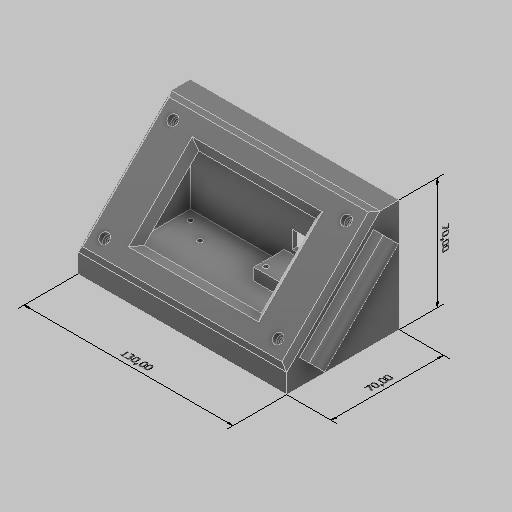
# Autodesk Inventor part: CASE - IHM
Saved by Autodesk Inventor 2025.2 (Build 292293000, 293)
## iProperties
Created: 2024-09-22
Part Number: CASE - IHM
Material: Genérico
Document SubType Name: Modeling
Designer: phmca
Density: 1 g/cm^3
Appearance: Suave - Preto
Author: phmca
Autodesk Inventor part; units mm, degrees
ref_plane "YZ Plane" through (0, 0, 0) normal (1, 0, 0) x (0, 1, 0)
ref_plane "XZ Plane" through (0, 0, 0) normal (0, 1, 0) x (-1, 0, 0)
sketch "Esboço1" plane through (0, 0, 0) normal (0, 1, 0) x (-1, 0, 0)
  line L0 (65, 35) -> (-65, 35)
  line L1 (-65, 35) -> (-65, -35)
  line L2 (-65, -35) -> (65, -35)
  line L3 (65, -35) -> (65, 35)
  point P0 (0, 0)
  dimension "d0" = 130
  dimension "d1" = 65
  dimension "d2" = 70
  dimension "d3" = 35
  constraints: 8 end point, 2 parallel, 1 horizontal, 1 perpendicular
  measures "d0" distance of L1.end L2.end
  measures "d1" distance from line of L3 point (0, 0)
  measures "d2" distance of L0.end L1.end
  measures "d3" distance from line of point (0, 0) L2
extrude "Extrusão1" add sketch "Esboço1" along normal blind 3
sketch "Esboço2" plane through (0, 3, 0) normal (0, 1, 0) x (1, 0, 0)
  line L0 (65, -35) -> (65, 35) projected
  line L1 (65, 35) -> (-65, 35) projected
  line L2 (-65, 35) -> (-65, -35) projected
  line L3 (-65, -35) -> (65, -35) projected
  line L4 (-62, 32) -> (62, 32)
  line L5 (62, 32) -> (62, -32)
  line L6 (62, -32) -> (-62, -32)
  line L7 (-62, -32) -> (-62, 32)
  point P0 (0, 0)
  dimension "d6" = 3
  dimension "d7" = 3
  dimension "d8" = 3
  dimension "d9" = 3
  constraints: 8 end point, 2 parallel, 1 horizontal, 1 perpendicular
  measures "d6" distance between parallel lines of L1 L4
  measures "d7" distance between parallel lines of L3 L6
  measures "d8" distance between parallel lines of L2 L7
  measures "d9" distance between parallel lines of L0 L5
extrude "Extrusão2" add sketch "Esboço2" along normal blind 67
sketch "Esboço3" plane through (-62, 3, 32) normal (1, 0, 0) x (0, 0, -1)
  line L0 (64, 0) -> (0, 0) projected
  line L1 (64, 0) -> (64, 67) projected
  line L2 (0, 67) -> (64, 67) projected
  line L3 (0, 0) -> (0, 67) projected
  line L4 (0, 64) -> (64, 64)
  point P0 (32, -3)
  dimension "d12" = 3
  constraints: 2 end point, 2 point on line, 1 perpendicular
  measures "d12" distance between parallel lines of L2 L4
extrude "Extrusão3" add sketch "Esboço3" along normal up to surface (124 mm away) contours L4 L3 L2 L1
sketch "Esboço4" plane through (65, 0, 35) normal (1, 0, 0) x (0, 0, -1)
  line L0 (0, 0) -> (0, 70) projected
  line L1 (0, 12) -> (58, 70)
  line L2 (70, 70) -> (0, 70) projected
  line L3 (0, 12) -> (0, 0) construction
  line L4 (58, 70) -> (70, 70) construction
  line L5 (67, 67) -> (3, 67) projected
  line L6 (70, 0) -> (70, 70) projected
  line L7 (58, 70) -> (70, 70)
  line L8 (0, 12) -> (0, 0)
  line L9 (0, 0) -> (70, 0) projected
  point P0 (35, 0)
  point P1 (55, 67)
  dimension "d15" = 45
  dimension "d20" = 3
  dimension "d21" = 4.2426
  dimension "d160" = 12
  dimension "d161" = 12
  constraints: 10 end point, 4 point on line, 3 collinear, 1 horizontal
  measures "d15" angle of L0 L1
  measures "d20" horizontal distance of L1.end point (55, 67)
  measures "d21" distance of L1.end point (55, 67)
  measures "d160" distance from line of L6 L1.end
  measures "d161" distance from line of L9 L1.start
extrude "Extrusão4" cut sketch "Esboço4" against normal up to surface (130 mm away) contours L0 L2 L1
sketch "Esboço6" plane through (-65, 12, 35) normal (0, 0.7071068, 0.7071068) x (1, 0, 0)
  line L0 (127, 77.7817) -> (3, 77.7817) projected
  line L1 (3, 77.7817) -> (3, 4.2426) projected
  line L2 (3, 4.2426) -> (127, 4.2426) projected
  line L3 (127, 4.2426) -> (127, 77.7817) projected
  line L4 (3, 77.7817) -> (11, 77.7817)
  line L5 (11, 77.7817) -> (11, 69.7817)
  line L6 (11, 69.7817) -> (3, 69.7817)
  line L7 (3, 69.7817) -> (3, 77.7817)
  line L8 (127, 77.7817) -> (119, 77.7817)
  line L9 (119, 77.7817) -> (119, 69.7817)
  line L10 (119, 69.7817) -> (127, 69.7817)
  line L11 (127, 69.7817) -> (127, 77.7817)
  line L12 (3, 4.2426) -> (11, 4.2426)
  line L13 (11, 4.2426) -> (11, 12.2426)
  line L14 (11, 12.2426) -> (3, 12.2426)
  line L15 (3, 12.2426) -> (3, 4.2426)
  line L16 (127, 4.2426) -> (119, 4.2426)
  line L17 (119, 4.2426) -> (119, 12.2426)
  line L18 (119, 12.2426) -> (127, 12.2426)
  line L19 (127, 12.2426) -> (127, 4.2426)
  point P0 (65, 16.2635)
  point P1 (119, 77.7817)
  point P2 (3, 12.2426)
  point P3 (11, 4.2426)
  point P4 (3, 69.7817)
  dimension "d31" = 8
  dimension "d32" = 8
  dimension "d33" = 8
  dimension "d34" = 8
  dimension "d35" = 8
  dimension "d36" = 8
  dimension "d37" = 8
  dimension "d38" = 8
  constraints: 32 end point, 8 parallel, 4 horizontal, 4 perpendicular
  measures "d31" distance of L5.end L6.end
  measures "d32" distance of L4.end L5.end
  measures "d33" distance of L10.end L9.end
  measures "d34" distance of L9.end L8.end
  measures "d35" distance of L14.end L13.end
  measures "d36" distance of L13.end L12.end
  measures "d37" distance of L17.end L18.end
  measures "d38" distance of L16.end L17.end
extrude "Extrusão6" [suppressed]
sketch "Esboço7" plane through (62, 3, -32) normal (-1, 0, 0) x (0, 0, 1)
  line L0 (64, 12) -> (12, 64) projected
  line L1 (12, 64) -> (0, 64) projected
  line L2 (0, 0) -> (0, 64) projected
  line L3 (64, 0) -> (0, 0) projected
  line L4 (64, 0) -> (64, 12) projected
  line L5 (12, 52.6863) -> (6.3431, 52.6863)
  line L6 (6.3431, 52.6863) -> (6.3431, 64)
  line L7 (58.3431, -13.6569) -> (65.4142, -13.6569)
  line L8 (58.3431, -13.6569) -> (52.6863, -13.6569)
  line L9 (52.6863, -13.6569) -> (52.6863, 2)
  point P0 (32, -3)
  point P1 (54, 6.3431)
  constraints: 10 end point, 3 horizontal, 2 perpendicular, 1 point on line
extrude "Extrusão7" [suppressed]
fillet "Arredondamento2" [suppressed]
sketch "Esboço8" plane through (62, 3, -32) normal (-1, 0, 0) x (0, 0, 1)
  line L0 (64, 12) -> (12, 64) projected
  line L1 (12, 64) -> (0, 64) projected
  line L2 (0, 0) -> (0, 64) projected
  line L3 (64, 0) -> (0, 0) projected
  line L4 (64, 0) -> (64, 12) projected
  line L5 (58.3431, 6.3431) -> (64, 6.3431)
  line L6 (6.3431, 58.3431) -> (6.3431, 64)
  point P0 (32, -3)
  constraints: 4 end point, 2 point on line, 1 perpendicular, 1 vertical
extrude "Extrusão8" [suppressed]
sketch "Esboço9" plane through (-62, 3, 32) normal (1, 0, 0) x (0, 0, -1)
  line L0 (0, 0) -> (0, 12) projected
  line L1 (64, 0) -> (0, 0) projected
  line L2 (64, 0) -> (64, 64) projected
  line L3 (64, 64) -> (52, 64) projected
  line L4 (52, 64) -> (0, 12) projected
  line L5 (57.6569, 58.3431) -> (57.6569, 64)
  line L6 (5.6569, 6.3431) -> (0, 6.3431)
  point P0 (32, -3)
  point P1 (0, 6.3431)
  constraints: 4 end point, 2 perpendicular, 1 point on line
extrude "Extrusão9" [suppressed]
sketch "Esboço10" plane through (65, 0, 35) normal (1, 0, 0) x (0, 0, -1)
  line L0 (67, 3) -> (3, 3) projected
  line L1 (3, 3) -> (67, 3) projected
  line L2 (67, 3) -> (67, 67) projected
  line L3 (67, 3) -> (67, 67) projected
  line L4 (26.8906, 26.9296) -> (53.3906, 26.9296)
  line L5 (53.3906, 26.9296) -> (53.3906, 5.4296)
  line L6 (53.3906, 5.4296) -> (26.8906, 5.4296)
  line L7 (26.8906, 5.4296) -> (26.8906, 26.9296)
  point P0 (35, 0)
  dimension "d48" = 26.5
  dimension "d49" = 21.5
  constraints: 8 end point, 2 parallel, 1 horizontal, 1 perpendicular
  measures "d48" distance of L4.start L4.end
  measures "d49" distance of L4.end L5.end
sketch "Esboço11" plane through (65, 0, -35) normal (0, 0, -1) x (-1, 0, 0)
  line L0 (127, 3) -> (3, 3) projected
  line L1 (3, 3) -> (127, 3) projected
  line L2 (3, 15) -> (3, 67) projected
  line L3 (3, 3) -> (3, 67) projected
  line L4 (13, 13) -> (39.5, 13)
  line L5 (39.5, 13) -> (39.5, 34.5)
  line L6 (39.5, 34.5) -> (13, 34.5)
  line L7 (13, 34.5) -> (13, 13)
  line L8 (51.5, 13) -> (63.6, 13)
  line L9 (63.6, 13) -> (63.6, 23.85)
  line L10 (63.6, 23.85) -> (51.5, 23.85)
  line L11 (51.5, 23.85) -> (51.5, 13)
  line L12 (3, 3) -> (3, 15) projected
  point P0 (65, 0)
  dimension "d50" = 26.5
  dimension "d51" = 21.5
  dimension "d52" = 10
  dimension "d53" = 10
  dimension "d67" = 12
  dimension "d68" = 12.1
  dimension "d69" = 10.85
  constraints: 16 end point, 4 parallel, 2 horizontal, 2 perpendicular, 1 collinear
  measures "d50" distance of L6.end L5.end
  measures "d51" distance of L5.end L4.end
  measures "d52" distance between parallel lines of L2 L7
  measures "d53" distance between parallel lines of L1 L4
  measures "d67" distance between parallel lines of L11 L5
  measures "d68" distance of L9.end L10.end
  measures "d69" distance between parallel lines of L8 L10
extrude "Extrusão10" cut sketch "Esboço11" against normal blind 28 contours L7 L6 L5 L4
sketch "Esboço12" plane through (-62, 3, -32) normal (0, 0, 1) x (1, 0, 0)
  line L0 (87.5, 31.5) -> (114, 31.5) projected
  line L1 (87.5, 10) -> (87.5, 31.5) projected
  line L2 (114, 10) -> (87.5, 10) projected
  line L3 (114, 31.5) -> (114, 10) projected
  line L4 (84.5, 34.5) -> (117, 34.5)
  line L5 (117, 34.5) -> (117, 7)
  line L6 (117, 7) -> (84.5, 7)
  line L7 (84.5, 7) -> (84.5, 34.5)
  point P0 (62, -3)
  dimension "d56" = 3
  dimension "d57" = 3
  dimension "d58" = 3
  dimension "d59" = 3
  constraints: 8 end point, 2 parallel, 1 horizontal, 1 perpendicular
  measures "d56" distance between parallel lines of L5 L3
  measures "d57" distance between parallel lines of L4 L0
  measures "d58" distance between parallel lines of L7 L1
  measures "d59" distance between parallel lines of L2 L6
extrude "Extrusão11" cut sketch "Esboço12" against normal blind 1.5
sketch "Esboço13" plane through (0, 3, 0) normal (0, 1, 0) x (1, 0, 0)
  line L0 (-62, 32) -> (-62, -32) projected
  line L1 (-62, -32) -> (62, -32) projected
  line L2 (62, -32) -> (62, 32) projected
  line L3 (62, 32) -> (-62, 32) projected
  line L4 (37, 3) -> (62, 3)
  line L5 (62, 3) -> (62, -32)
  line L6 (62, -32) -> (27, -32)
  line L7 (27, -32) -> (27, -7)
  arc A0 (37, 3) -> (27, -7) centre (37, -7) ccw
  point P0 (0, 0)
  point P1 (27, 3)
  point P2 (27, -32)
  dimension "d62" = 35
  dimension "d63" = 35
  dimension "d64" = 10
  constraints: 8 end point, 2 collinear, 2 parallel, 2 point on circle, 2 point on line, 2 tangent, 1 centre point, 1 horizontal, 1 perpendicular
  measures "d62" distance of point (27, 3) L4.end
  measures "d63" distance of L6.end point (27, 3)
  measures "d64" radius of A0
extrude "Extrusão12" cut sketch "Esboço13" against normal up to surface (3 mm away) contours L7 A0 L4 L2 L1
extrude "Extrusão13" cut sketch "Esboço11" against normal up to surface (3 mm away) contours L11 L10 L9 L8
sketch "Esboço14" plane through (0, 3, 0) normal (0, 1, 0) x (1, 0, 0)
  line L0 (13.5, 35) -> (1.4, 35) projected
  line L1 (-3.55, 13) -> (18.45, 13)
  line L2 (18.45, 13) -> (18.45, 35)
  line L3 (18.45, 35) -> (-3.55, 35)
  line L4 (-3.55, 35) -> (-3.55, 13)
  circle A0 centre (0, 17) radius 1.45
  circle A1 centre (14.9, 17) radius 1.45
  line L5 (0, 17) -> (-3.55, 17) construction
  line L6 (14.9, 17) -> (18.45, 17) construction
  point P0 (0, 0)
  point P1 (7.45, 35)
  dimension "d72" = 22
  dimension "d73" = 22
  dimension "d74" = 2.9
  dimension "d75" = 2.9
  dimension "d76" = 14.9
  dimension "d78" = 18
  dimension "d79" = 11
  dimension "d216" = 4
  constraints: 12 end point, 3 collinear, 3 perpendicular, 2 centre point, 2 parallel, 2 point on line, 1 horizontal, 1 midpoint
  measures "d72" distance of L1.start L1.end
  measures "d73" distance of L3.end L1.start
  measures "d74" diameter of A0
  measures "d75" diameter of A1
  measures "d76" distance of L6.start L5.start
  measures "d78" distance between parallel lines of L3 L5
  measures "d79" distance from line of L4 point (7.45, 35)
  measures "d216" distance from line of L1 L5.start
extrude "Extrusão14" add sketch "Esboço14" along normal blind 7.5 contours L3 L2 L1 L4 L0 | A0 | A1
sketch "Esboço15" plane through (0, 10.5, 0) normal (0, 1, 0) x (1, 0, 0)
  circle A0 centre (0, 17) radius 1.45 projected
  circle A1 centre (14.9, 17) radius 1.45 projected
  point P0 (0, 0)
extrude "Extrusão15" cut sketch "Esboço15" against normal blind 9
sketch "Esboço16" plane through (-65, 12, 35) normal (0, 0.7071068, 0.7071068) x (1, 0, 0)
  line L0 (127, 4.2426) -> (127, 77.7817) projected
  line L1 (3, 4.2426) -> (127, 4.2426) projected
  line L2 (3, 77.7817) -> (3, 4.2426) projected
  line L3 (127, 77.7817) -> (3, 77.7817) projected
  line L4 (0, 0) -> (0, 82.0244) projected
  line L5 (130, 0) -> (0, 0) projected
  line L6 (130, 82.0244) -> (130, 0) projected
  line L7 (0, 82.0244) -> (130, 82.0244) projected
  circle A0 centre (6, 7.2426) radius 1.45
  circle A1 centre (6, 74.7817) radius 1.45
  circle A2 centre (124, 74.7817) radius 1.45
  circle A3 centre (124, 7.2426) radius 1.45
  point P0 (65, 16.2635)
  dimension "d84" = 2.9
  dimension "d85" = 2.9
  dimension "d86" = 2.9
  dimension "d87" = 2.9
  constraints: 4 centre point
  measures "d84" diameter of A0
  measures "d85" diameter of A1
  measures "d86" diameter of A2
  measures "d87" diameter of A3
extrude "Extrusão16" [suppressed]
sketch "Esboço17" plane through (0, 3, 0) normal (0, 1, 0) x (1, 0, 0)
  line L0 (-3.55, 32) -> (-62, 32) projected
  line L1 (-62, 32) -> (-62, -32) projected
  line L2 (-62, -32) -> (27, -32) projected
  line L3 (62, 3) -> (62, 32) projected
  circle A0 centre (-56, 26) radius 1.55
  circle A1 centre (-56, -12) radius 1.55
  circle A2 centre (21, -26) radius 1.55
  circle A3 centre (56, 9) radius 1.55
  circle A4 centre (56, 26) radius 1.55
  line L4 (37, 3) -> (62, 3) projected
  line L5 (27, -32) -> (27, -7) projected
  arc A5 (37, 3) -> (27, -7) centre (37, -7) ccw projected
  line L6 (-3.55, 13) -> (-3.55, 32) projected
  line L7 (62, 32) -> (18.45, 32) projected
  line L8 (18.45, 32) -> (18.45, 13) projected
  line L9 (18.45, 13) -> (-3.55, 13) projected
  circle A6 centre (-42, -26) radius 1.55
  circle A7 centre (-42, -12) radius 1.55
  circle A8 centre (21, -12) radius 1.55
  circle A9 centre (21, 18) radius 1.55
  circle A10 centre (-42, 18) radius 1.55
  point P0 (0, 0)
  dimension "d90" = 3.1
  dimension "d91" = 3.1
  dimension "d92" = 3.1
  dimension "d93" = 3.1
  dimension "d94" = 3.1
  dimension "d95" = 6
  dimension "d96" = 6
  dimension "d97" = 6
  dimension "d98" = 20
  dimension "d100" = 6
  dimension "d102" = 6
  dimension "d104" = 6
  dimension "d157" = 6
  dimension "d158" = 6
  dimension "d159" = 6
  dimension "d207" = 3.1
  dimension "d208" = 20
  dimension "d209" = 6
  dimension "d217" = 3.1
  dimension "d218" = 3.1
  dimension "d219" = 3.1
  dimension "d220" = 3.1
  dimension "d221" = 20
  dimension "d222" = 20
  dimension "d223" = 20
  dimension "d224" = 6
  dimension "d225" = 50
  dimension "d226" = 6
  dimension "d227" = 50
  dimension "d228" = 20
  constraints: 10 centre point
  measures "d90" diameter of A0
  measures "d91" diameter of A1
  measures "d92" diameter of A2
  measures "d93" diameter of A3
  measures "d94" diameter of A4
  measures "d95" distance from line of L1 A0.centre
  measures "d96" distance from line of L0 A0.centre
  measures "d97" distance from line of L1 A1.centre
  measures "d98" distance from line of L2 A1.centre
  measures "d100" distance from line of L2 A2.centre
  measures "d102" distance from line of L3 A3.centre
  measures "d104" distance from line of L3 A4.centre
  measures "d157" distance from line of L7 A4.centre
  measures "d158" distance from line of L4 A3.centre
  measures "d159" distance from line of L5 A2.centre
  measures "d207" diameter of A6
  measures "d208" distance from line of L1 A6.centre
  measures "d209" distance from line of L2 A6.centre
  measures "d217" diameter of A7
  measures "d218" diameter of A8
  measures "d219" diameter of A9
  measures "d220" diameter of A10
  measures "d221" distance from line of L1 A7.centre
  measures "d222" distance from line of L2 A8.centre
  measures "d223" distance from line of L2 A7.centre
  measures "d224" distance from line of L5 A8.centre
  measures "d225" distance from line of L2 A9.centre
  measures "d226" distance from line of L5 A9.centre
  measures "d227" distance from line of L2 A10.centre
  measures "d228" distance from line of L1 A10.centre
extrude "Extrusão17" cut sketch "Esboço17" against normal up to surface (3 mm away) contours A0 | A1 | A2 | A3 | A4 | A6 | A7 | A8 | A9 | A10
sketch "Esboço18" plane through (65, 0, 35) normal (1, 0, 0) x (0, 0, -1)
  line L0 (58, 70) -> (0, 12) projected
  line L1 (58, 70) -> (53.7574, 70)
  line L2 (53.7574, 70) -> (0, 16.2426)
  line L3 (0, 16.2426) -> (0, 12)
  point P0 (35, 0)
  dimension "d107" = 3
  constraints: 6 end point, 2 perpendicular, 1 horizontal
  measures "d107" distance between parallel lines of L0 L2
extrude "Extrusão18" add sketch "Esboço18" against normal up to surface (130 mm away) separate body
chamfer "Chanfro1" distance 3 angle 45 2 edges at (65, 43.1213, 8.1213) (-65, 43.1213, 8.1213)
sketch "Esboço19" plane through (65, 70, -23) normal (0, -0.7071068, -0.7071068) x (-1, 0, 0)
  circle A0 centre (6, -7.2426) radius 1.45 projected
  circle A1 centre (124, -7.2426) radius 1.45 projected
  circle A2 centre (124, -74.7817) radius 1.45 projected
  circle A3 centre (6, -74.7817) radius 1.45 projected
  circle A4 centre (124, -74.7817) radius 1.75
  circle A5 centre (6, -74.7817) radius 1.75
  circle A6 centre (124, -7.2426) radius 1.75
  circle A7 centre (6, -7.2426) radius 1.75
  point P0 (65, -65.7609)
  dimension "d115" = 3.5
  dimension "d116" = 3.5
  dimension "d117" = 3.5
  dimension "d118" = 3.5
  constraints: 4 centre point, 4 coincident
  measures "d115" diameter of A4
  measures "d116" diameter of A5
  measures "d117" diameter of A6
  measures "d118" diameter of A7
extrude "Extrusão19" [suppressed]
sketch "Esboço20" plane through (65, 70, -23) normal (0, -0.7071068, -0.7071068) x (-1, 0, 0)
  line L0 (125, -77.0244) -> (5, -77.0244)
  line L1 (5, -77.0244) -> (5, -5)
  line L2 (5, -5) -> (125, -5)
  line L3 (125, -5) -> (125, -77.0244)
  line L4 (130, -82.0244) -> (130, 0) projected
  line L5 (0, 0) -> (130, 0) projected
  line L6 (0, -82.0244) -> (0, 0) projected
  line L7 (0, -82.0244) -> (130, -82.0244) projected
  point P0 (65, -65.7609)
  dimension "d119" = 5
  dimension "d120" = 5
  dimension "d121" = 5
  dimension "d122" = 5
  constraints: 8 end point, 2 parallel, 1 horizontal, 1 perpendicular
  measures "d119" distance between parallel lines of L7 L0
  measures "d120" distance between parallel lines of L4 L3
  measures "d121" distance between parallel lines of L5 L2
  measures "d122" distance between parallel lines of L6 L1
extrude "Extrusão20" add sketch "Esboço20" along normal blind 1 contours L0 L1 L2 L3 bodies 2
sketch "Esboço21" plane through (65, 69.2929, -23.7071) normal (0, -0.7071068, -0.7071068) x (-1, 0, 0)
  line L0 (125, -5) -> (125, -77.0244) projected
  line L1 (125, -77.0244) -> (5, -77.0244) projected
  line L2 (5, -77.0244) -> (5, -5) projected
  line L3 (5, -5) -> (125, -5) projected
  line L4 (130, -82.0244) -> (130, 0) projected
  line L5 (0, 0) -> (130, 0) projected
  line L6 (0, -82.0244) -> (0, 0) projected
  line L7 (0, -82.0244) -> (130, -82.0244) projected
  line L8 (28.5, -17.0122) -> (101.5, -17.0122)
  line L9 (101.5, -17.0122) -> (101.5, -65.0122)
  line L10 (101.5, -65.0122) -> (28.5, -65.0122)
  line L11 (28.5, -65.0122) -> (28.5, -17.0122)
  point P0 (65, -65.7609)
  point P1 (65, -17.0122)
  point P2 (28.5, -41.0122)
  dimension "d125" = 73
  dimension "d126" = 48
  dimension "d127" = 130
  dimension "d128" = 65
  dimension "d129" = 82.0244
  dimension "d130" = 41.0122
  constraints: 8 end point, 2 midpoint, 2 parallel, 1 horizontal, 1 perpendicular
  measures "d125" distance of L9.end L10.end
  measures "d126" distance of L8.end L9.end
  measures "d127" distance between parallel lines of L6 L4
  measures "d128" distance from line of L6 point (65, -17.012)
  measures "d129" distance of L6.start L5.start
  measures "d130" distance from line of L7 point (28.5, -41.012)
extrude "Extrusão21" cut sketch "Esboço21" against normal up to surface (4 mm away) contours L8 L9 L10 L11 bodies 2
sketch "Esboço22" plane through (65, 69.2929, -23.7071) normal (0, -0.7071068, -0.7071068) x (-1, 0, 0)
  line L0 (115, -16.7422) -> (115, -65.2822) construction
  line L1 (20.9, -65.2822) -> (20.9, -16.7422) construction
  line L2 (125, -5) -> (125, -77.0244) construction
  line L3 (125, -77.0244) -> (5, -77.0244) construction
  line L4 (5, -77.0244) -> (5, -5) construction
  line L5 (5, -5) -> (125, -5) construction
  line L6 (130, -82.0244) -> (130, 0) construction
  line L7 (0, 0) -> (130, 0) construction
  line L8 (0, -82.0244) -> (0, 0) construction
  line L9 (0, -82.0244) -> (130, -82.0244) construction
  circle A0 centre (20.9, -16.7422) radius 1.45
  circle A1 centre (20.9, -16.7422) radius 3
  circle A2 centre (115, -16.7422) radius 1.45
  circle A3 centre (115, -16.7422) radius 2.5
  circle A4 centre (20.9, -65.2822) radius 1.45
  circle A5 centre (20.9, -65.2822) radius 3
  circle A6 centre (115, -65.2822) radius 1.45
  circle A7 centre (115, -65.2822) radius 2.5
  line L10 (18.9, -18.9783) -> (22.9, -18.9783) construction
  line L11 (22.9, -18.9783) -> (22.9, -63.0461)
  line L12 (22.9, -63.0461) -> (18.9, -63.0461) construction
  line L13 (18.9, -63.0461) -> (18.9, -18.9783)
  line L14 (113, -18.2422) -> (117, -18.2422) construction
  line L15 (117, -18.2422) -> (117, -63.7822)
  line L16 (117, -63.7822) -> (113, -63.7822) construction
  line L17 (113, -63.7822) -> (113, -18.2422)
  line L18 (20.9, -65.2822) -> (115, -65.2822)
  line L19 (20.9, -16.7422) -> (115, -16.7422)
  point P0 (65, -65.7609)
  point P1 (20.9, -41.0122)
  point P2 (65, -16.2822)
  point P3 (113, -18.2422)
  point P4 (113, -63.7822)
  point P5 (18.9, -18.9783)
  dimension "d140" = 6
  dimension "d142" = 5
  dimension "d144" = 6
  dimension "d146" = 5
  dimension "d134" = 48.54
  dimension "d135" = 82.0244
  dimension "d136" = 130
  dimension "d137" = 41.0122
  dimension "d139" = 2.9
  dimension "d141" = 2.9
  dimension "d143" = 2.9
  dimension "d145" = 2.9
  dimension "d151" = 4
  dimension "d152" = 2
  dimension "d153" = 4
  dimension "d154" = 2
  dimension "d241" = 44.1
  dimension "d243" = 50
  constraints: 24 end point, 8 coincident, 5 parallel, 4 centre point, 4 perpendicular, 2 horizontal, 1 midpoint, 12 other
  measures "d134" distance of L1.start L1.end
  measures "d135" distance of L8.start L7.start
  measures "d136" distance of L7.start L6.end
  measures "d137" vertical distance of L7.start point (20.9, -41.012)
  measures "d139" diameter of A0
  measures "d141" diameter of A2
  measures "d143" diameter of A4
  measures "d145" diameter of A6
  measures "d151" distance of L11.end L12.end
  measures "d152" distance between parallel lines of L13 L1
  measures "d153" distance of L15.end L16.end
  measures "d154" distance between parallel lines of L0 L17
  measures "d241" distance from line of point (65, -16.282) L1
  measures "d243" distance from line of L0 point (65, -16.282)
extrude "Extrusão22" add sketch "Esboço22" along normal blind 3.7 contours A1 | A3 | A5 | A7 bodies 2
extrude "Extrusão23" cut sketch "Esboço22" against normal blind 3.3 contours A0 | A2 | A4 | A6 bodies 2
extrude "Extrusão24" add sketch "Esboço22" along normal blind 3 contours A1 L11 A5 L13 | A3 L15 A7 L17 bodies 2
sketch "Esboço23" plane through (-62, 16.2426, 35) normal (0, 0.7071068, 0.7071068) x (1, 0, 0)
  circle A0 centre (8, 68.0244) radius 3
  circle A1 centre (8, 68.0244) radius 1.75
  circle A2 centre (116, 68.0244) radius 1.75
  circle A3 centre (116, 68.0244) radius 3
  circle A4 centre (116, 8) radius 1.75
  circle A5 centre (116, 8) radius 3
  circle A6 centre (8, 8) radius 1.75
  circle A7 centre (8, 8) radius 3
  line L0 (98.5, 62.0122) -> (98.5, 14.0122) projected
  line L1 (98.5, 14.0122) -> (25.5, 14.0122) projected
  line L2 (25.5, 14.0122) -> (25.5, 62.0122) projected
  line L3 (25.5, 62.0122) -> (98.5, 62.0122) projected
  line L4 (0, 0) -> (0, 76.0244) projected
  line L5 (124, 0) -> (0, 0) projected
  line L6 (124, 76.0244) -> (124, 0) projected
  line L7 (124, 76.0244) -> (0, 76.0244) projected
  point P0 (62, 13.2635)
  dimension "d162" = 6
  dimension "d163" = 3.5
  dimension "d164" = 3.5
  dimension "d165" = 6
  dimension "d166" = 3.5
  dimension "d167" = 6
  dimension "d168" = 3.5
  dimension "d169" = 6
  dimension "d170" = 8
  dimension "d171" = 8
  dimension "d172" = 8
  dimension "d173" = 8
  dimension "d174" = 8
  dimension "d175" = 8
  dimension "d176" = 8
  dimension "d177" = 8
  constraints: 8 centre point, 4 coincident
  measures "d162" diameter of A0
  measures "d163" diameter of A1
  measures "d164" diameter of A2
  measures "d165" diameter of A3
  measures "d166" diameter of A4
  measures "d167" diameter of A5
  measures "d168" diameter of A6
  measures "d169" diameter of A7
  measures "d170" distance from line of L4 A0.centre
  measures "d171" distance from line of L7 A0.centre
  measures "d172" distance from line of L7 A2.centre
  measures "d173" distance from line of L6 A2.centre
  measures "d174" distance from line of L5 A4.centre
  measures "d175" distance from line of L6 A4.centre
  measures "d176" distance from line of L5 A6.centre
  measures "d177" distance from line of L4 A7.centre
extrude "Extrusão25" cut sketch "Esboço23" against normal blind 3.5 contours A0 | A1 | A2 | A3 | A4 | A5 | A6 | A7 bodies 2
sketch "Esboço24" plane through (65, 69.2929, -23.7071) normal (0, -0.7071068, -0.7071068) x (-1, 0, 0)
  circle A0 centre (119, -71.0244) radius 1.75 projected
  circle A1 centre (119, -71.0244) radius 3 projected
  circle A2 centre (119, -11) radius 1.75 projected
  circle A3 centre (119, -11) radius 3 projected
  circle A4 centre (11, -11) radius 1.75 projected
  circle A5 centre (11, -11) radius 3 projected
  circle A6 centre (11, -71.0244) radius 1.75 projected
  circle A7 centre (11, -71.0244) radius 3 projected
  line L0 (125, -77.0244) -> (125, -5) projected
  line L1 (125, -77.0244) -> (115, -77.0244)
  line L2 (115, -77.0244) -> (115, -70.0244)
  line L3 (118, -67.0244) -> (125, -67.0244)
  line L4 (125, -67.0244) -> (125, -77.0244)
  arc A8 (118, -67.0244) -> (115, -70.0244) centre (118, -70.0244) ccw
  line L5 (5, -77.0244) -> (5, -5) projected
  line L6 (5, -77.0244) -> (15, -77.0244)
  line L7 (15, -77.0244) -> (15, -70.0244)
  line L8 (12, -67.0244) -> (5, -67.0244)
  line L9 (5, -67.0244) -> (5, -77.0244)
  line L10 (125, -5) -> (5, -5) projected
  line L11 (5, -5) -> (15, -5)
  line L12 (15, -5) -> (15, -12)
  line L13 (12, -15) -> (5, -15)
  line L14 (5, -15) -> (5, -5)
  line L15 (125, -5) -> (115, -5)
  line L16 (115, -5) -> (115, -12)
  line L17 (118, -15) -> (125, -15)
  line L18 (125, -15) -> (125, -5)
  arc A9 (115, -12) -> (118, -15) centre (118, -12) ccw
  arc A10 (12, -15) -> (15, -12) centre (12, -12) ccw
  arc A11 (15, -70.0244) -> (12, -67.0244) centre (12, -70.0244) ccw
  point P0 (65, -65.7609)
  point P1 (115, -67.0244)
  point P2 (15, -67.0244)
  point P3 (15, -15)
  point P4 (115, -15)
  point P5 (125, -15)
  point P6 (115, -5)
  point P7 (15, -5)
  point P8 (5, -15)
  dimension "d182" = 10
  dimension "d183" = 10
  dimension "d184" = 3
  dimension "d185" = 10
  dimension "d186" = 10
  dimension "d187" = 10
  dimension "d188" = 10
  dimension "d189" = 10
  dimension "d190" = 10
  dimension "d191" = 3
  dimension "d192" = 3
  dimension "d193" = 3
  constraints: 32 end point, 8 parallel, 8 point on circle, 8 point on line, 8 tangent, 4 centre point, 4 horizontal, 4 perpendicular
  measures "d182" distance of point (115, -67.024) L3.end
  measures "d183" distance of L1.end point (115, -67.024)
  measures "d184" radius of A8
  measures "d185" distance of point (15, -15) L13.end
  measures "d186" distance of L11.end point (15, -15)
  measures "d187" distance of L17.end point (115, -15)
  measures "d188" distance of point (115, -15) L15.end
  measures "d189" distance of point (15, -67.024) L8.end
  measures "d190" distance of L6.end point (15, -67.024)
  measures "d191" radius of A9
  measures "d192" radius of A10
  measures "d193" radius of A11
extrude "Extrusão27" add sketch "Esboço24" along normal blind 1 contours A0 | A1 | A2 | A3 | A4 | A5 | A6 | A7 | L1 L2 A8 L3 L0 | L17 A9 L16 L10 L0 | L5 L8 A11 L7 L6 | L5 L10 L12 A10 L13 bodies 2
extrude "Extrusão26" cut sketch "Esboço23" against normal through all contours A1 | A2 | A4 | A6 bodies 2
chamfer "Chanfro2" distance 4 angle 45 4 edges at (36.5, 43.1213, 8.1213) (0, 60.0919, -8.8492) (-36.5, 43.1213, 8.1213) (0, 26.1508, 25.0919)
sketch "Esboço25" plane through (65, 68.5858, -24.4142) normal (0, -0.7071068, -0.7071068) x (-1, 0, 0)
  circle A0 centre (119, -71.0244) radius 1.75 projected
  line L0 (125, -77.0244) -> (125, -67.0244) projected
  line L1 (125, -67.0244) -> (118, -67.0244) projected
  arc A1 (118, -67.0244) -> (115, -70.0244) centre (118, -70.0244) ccw projected
  line L2 (115, -70.0244) -> (115, -77.0244) projected
  line L3 (115, -77.0244) -> (125, -77.0244) projected
  circle A2 centre (119, -11) radius 1.75 projected
  line L4 (118, -15) -> (125, -15) projected
  line L5 (125, -15) -> (125, -5) projected
  line L6 (125, -5) -> (115, -5) projected
  line L7 (115, -5) -> (115, -12) projected
  arc A3 (115, -12) -> (118, -15) centre (118, -12) ccw projected
  line L8 (15, -5) -> (5, -5) projected
  circle A4 centre (11, -71.0244) radius 1.75 projected
  line L9 (12, -67.0244) -> (5, -67.0244) projected
  line L10 (5, -67.0244) -> (5, -77.0244) projected
  line L11 (5, -77.0244) -> (15, -77.0244) projected
  line L12 (15, -77.0244) -> (15, -70.0244) projected
  arc A5 (15, -70.0244) -> (12, -67.0244) centre (12, -70.0244) ccw projected
  circle A6 centre (11, -11) radius 1.75 projected
  line L13 (15, -12) -> (15, -5) projected
  line L14 (15, -5) -> (5, -5) projected
  line L15 (5, -5) -> (5, -15) projected
  line L16 (5, -15) -> (12, -15) projected
  arc A7 (12, -15) -> (15, -12) centre (12, -12) ccw projected
  circle A8 centre (119, -11) radius 1.45
  circle A9 centre (11, -11) radius 1.45
  circle A10 centre (11, -71.0244) radius 1.45
  circle A11 centre (119, -71.0244) radius 1.45
  point P0 (65, -65.7609)
  point P1 (15, -5)
  point P2 (5, -5)
  dimension "d210" = 2.9
  dimension "d211" = 2.9
  dimension "d212" = 2.9
  dimension "d213" = 2.9
  constraints: 4 centre point, 4 coincident
  measures "d210" diameter of A8
  measures "d211" diameter of A9
  measures "d212" diameter of A10
  measures "d213" diameter of A11
extrude "Extrusão28" add sketch "Esboço25" along normal blind 10 contours A0 | L3 L2 A1 L1 L0 | A2 | A3 L7 L6 L5 L4 | L13 A7 L16 L15 L8 | A4 | A5 L12 L11 L10 L9 | A6 | A8 | A9 | A10 | A11 bodies 1
sketch "Esboço26" plane through (65, 68.5858, -24.4142) normal (0, 0.7071068, 0.7071068) x (1, 0, 0)
  line L0 (-125, -67.0244) -> (-118, -67.0244) projected
  line L1 (-125, -77.0244) -> (-125, -67.0244) projected
  line L2 (-115, -77.0244) -> (-125, -77.0244) projected
  line L3 (-115, -70.0244) -> (-115, -77.0244) projected
  arc A0 (-115, -70.0244) -> (-118, -67.0244) centre (-118, -70.0244) ccw projected
  line L4 (-125, -15) -> (-125, -5) projected
  line L5 (-118, -15) -> (-125, -15) projected
  arc A1 (-118, -15) -> (-115, -12) centre (-118, -12) ccw projected
  line L6 (-115, -5) -> (-115, -12) projected
  line L7 (-125, -5) -> (-115, -5) projected
  line L8 (-15, -5) -> (-5, -5) projected
  line L9 (-15, -12) -> (-15, -5) projected
  arc A2 (-15, -12) -> (-12, -15) centre (-12, -12) ccw projected
  line L10 (-5, -15) -> (-12, -15) projected
  line L11 (-5, -5) -> (-5, -15) projected
  line L12 (-127, -4.2426) -> (-127, -77.7817) projected
  line L13 (-3, -77.7817) -> (-3, -4.2426) projected
  line L14 (-5, -67.0244) -> (-5, -77.0244) projected
  line L15 (-12, -67.0244) -> (-5, -67.0244) projected
  arc A3 (-12, -67.0244) -> (-15, -70.0244) centre (-12, -70.0244) ccw projected
  line L16 (-15, -77.0244) -> (-15, -70.0244) projected
  line L17 (-5, -77.0244) -> (-15, -77.0244) projected
  line L18 (-125, -15) -> (-127, -15)
  line L19 (-125, -5) -> (-127, -5)
  line L20 (-125, -67.0244) -> (-127, -67.0244)
  line L21 (-125, -77.0244) -> (-127, -77.0244)
  line L22 (-5, -77.0244) -> (-3, -77.0244)
  line L23 (-5, -67.0244) -> (-3, -67.0244)
  line L24 (-5, -15) -> (-3, -15)
  line L25 (-5, -5) -> (-5, -15) projected
  line L26 (-5, -5) -> (-3, -5)
  point P0 (-65, -65.7609)
  constraints: 16 end point, 8 point on line, 7 perpendicular, 1 parallel
extrude "Extrusão29" add sketch "Esboço26" against normal up to surface (10 mm away) contours L1 L21 L12 L20 | L18 L12 L19 L4 | L26 L13 L24 L11 | L22 L14 L23 L13 bodies 1
sketch "Esboço27" plane through (62, 3, -32) normal (-1, 0, 0) x (0, 0, 1)
  line L0 (47.9081, 11.1213) -> (54.9792, 18.1924) projected
  line L1 (54.9792, 18.1924) -> (62.0503, 11.1213) projected
  line L2 (62.0503, 11.1213) -> (54.9792, 4.0503) projected
  line L3 (54.9792, 4.0503) -> (47.9081, 11.1213) projected
  line L4 (18.1924, 54.9792) -> (11.1213, 47.9081) projected
  line L5 (11.1213, 47.9081) -> (4.0503, 54.9792) projected
  line L6 (4.0503, 54.9792) -> (11.1213, 62.0503) projected
  line L7 (11.1213, 62.0503) -> (18.1924, 54.9792) projected
  line L8 (64, 12) -> (12, 64) projected
  line L9 (12, 64) -> (0, 64) projected
  line L10 (0, 0) -> (0, 64) projected
  line L11 (29, 0) -> (0, 0) projected
  line L12 (29, 0) -> (29, -3) projected
  line L13 (64, -3) -> (29, -3) projected
  line L14 (64, 12) -> (64, -3) projected
  line L15 (54.9792, 4.0503) -> (64, 4.5)
  line L16 (62.0503, 11.1213) -> (64, 9.1716)
  line L17 (11.1213, 62.0503) -> (9.1716, 64)
  line L18 (4.0503, 54.9792) -> (4.0503, 64)
  point P0 (32, -3)
  constraints: 8 end point, 3 point on line, 2 perpendicular, 1 collinear, 1 midpoint
extrude "Extrusão30" add sketch "Esboço27" along normal up to surface (12 mm away) contours L2 L16 L14 L15 | L17 L6 L18 L9 bodies 1
sketch "Esboço28" plane through (-62, 3, 32) normal (1, 0, 0) x (0, 0, -1)
  line L0 (45.8076, 54.9792) -> (52.8787, 62.0503) projected
  line L1 (52.8787, 62.0503) -> (59.9497, 54.9792) projected
  line L2 (59.9497, 54.9792) -> (52.8787, 47.9081) projected
  line L3 (52.8787, 47.9081) -> (45.8076, 54.9792) projected
  line L4 (1.9497, 11.1213) -> (9.0208, 18.1924) projected
  line L5 (9.0208, 18.1924) -> (16.0919, 11.1213) projected
  line L6 (16.0919, 11.1213) -> (9.0208, 4.0503) projected
  line L7 (9.0208, 4.0503) -> (1.9497, 11.1213) projected
  line L8 (52, 64) -> (0, 12) projected
  line L9 (0, 0) -> (0, 12) projected
  line L10 (64, 0) -> (0, 0) projected
  line L11 (64, 0) -> (64, 64) projected
  line L12 (64, 64) -> (52, 64) projected
  line L13 (1.9497, 11.1213) -> (0, 9.1716)
  line L14 (9.0208, 4.0503) -> (0, 4.0503)
  line L15 (59.9497, 54.9792) -> (59.9497, 64)
  line L16 (52.8787, 62.0503) -> (54.8284, 64)
  point P0 (32, -3)
  constraints: 8 end point, 4 point on line, 3 perpendicular, 1 collinear
extrude "Extrusão31" add sketch "Esboço28" along normal up to surface (12 mm away) contours L16 L12 L15 L1 | L13 L7 L14 L9 bodies 1
extrude "Extrusão32" cut sketch "Esboço25" along normal blind 9 contours A8 | A9 | A10 | A11 bodies 1
sketch "Esboço29" plane through (65, 0, 35) normal (1, 0, 0) x (0, 0, -1)
  line L0 (8.0381, 16) -> (54, 61.9619)
  line L1 (70, 0) -> (70, 70) projected
  line L2 (0, 0) -> (70, 0) projected
  line L3 (8.0381, 16) -> (15.1091, 8.9289)
  line L4 (15.1091, 8.9289) -> (61.0711, 54.8909)
  line L5 (61.0711, 54.8909) -> (54, 61.9619)
  line L6 (58, 70) -> (0, 12) projected
  line L7 (8.0381, 16) -> (8.0381, 0) construction
  line L8 (54, 61.9619) -> (70, 61.9619) construction
  line L9 (8.0381, 16) -> (0.967, 8.9289)
  line L10 (0.967, 8.9289) -> (8.0381, 1.8579)
  line L11 (8.0381, 1.8579) -> (15.1091, 8.9289)
  line L12 (61.0711, 54.8909) -> (68.1421, 61.9619)
  line L13 (52.6613, 61.8329) -> (59.0253, 55.469) projected
  line L14 (68.1421, 61.9619) -> (61.0711, 69.033)
  line L15 (61.0711, 69.033) -> (54, 61.9619)
  point P0 (35, 0)
  dimension "d229" = 65
  dimension "d230" = 45
  dimension "d231" = 10
  dimension "d232" = 16
  dimension "d233" = 10
  dimension "d234" = 10
  constraints: 24 end point, 11 perpendicular, 2 point on line
  measures "d229" distance of L0.start L0.end
  measures "d230" angle of L2 L0
  measures "d231" distance of L0.start L3.end
  measures "d232" distance of L0.end L8.end
  measures "d233" distance of L0.start L9.end
  measures "d234" distance of L14.end L0.end
extrude "Extrusão33" add sketch "Esboço29" along normal blind 1 separate body contours L0 L5 L4 L3
ref_plane "Plano de trabalho1" through (66, 61.9619, -19) normal (0, -0.7071068, 0.7071068) x (1, 0, 0)
sketch "Esboço30" plane through (66, 61.9619, -19) normal (0, -0.7071068, 0.7071068) x (1, 0, 0)
  arc A0 (5, -10) -> (5, 0) centre (5, -5) ccw
  line L0 (-1, 0) -> (0, 0) projected
  line L1 (0, -10) -> (0, 0) projected
  circle A1 centre (5, -5) radius 4.5
  line L2 (0, 0) -> (5, 0)
  line L3 (0, -10) -> (5, -10)
  point P0 (-66, -30.3787)
  dimension "d237" = 10
  dimension "d238" = 9
  constraints: 4 end point, 3 tangent, 2 centre point, 2 point on circle, 1 coincident, 1 horizontal
  measures "d237" diameter of A0
  measures "d238" diameter of A1
extrude "Extrusão34" add sketch "Esboço30" along normal up to surface (65 mm away) separate body
combine bodies "Combinar1" operation type add bodies to combine 3 4
sketch "Esboço31" plane through (65, 69.2929, -23.7071) normal (0, -0.7071068, -0.7071068) x (-1, 0, 0)
  line L0 (101.5, -65.0122) -> (28.5, -65.0122) projected
  line L1 (65, -65.0122) -> (65, -17.0122)
  line L2 (28.5, -17.0122) -> (101.5, -17.0122) projected
  line L3 (28.5, -65.0122) -> (28.5, -17.0122) projected
  line L4 (28.5, -41.0122) -> (101.5, -41.0122)
  line L5 (101.5, -17.0122) -> (101.5, -65.0122) projected
  circle A0 centre (65, -41.0122) radius 6.03
  point P0 (65, -65.7609)
  constraints: 5 midpoint, 4 end point, 1 centre point
equation "\"d1\" = 0.5 * d0"
equation "\"d3\" = 0.5 * d2"
equation "\"d7\" = d6"
equation "\"d79\" = 0.5 * d72"
equation "\"d97\" = d95"
equation "\"d100\" = d95"
equation "\"d157\" = d158"
equation "\"d158\" = d159"
equation "\"d159\" = d100"
equation "\"d120\" = d119"
equation "\"d121\" = d119"
equation "\"d122\" = d119"
equation "\"d130\" = 0.5 * d129"
equation "\"d137\" = 0.5 * d135"
equation "\"d152\" = 0.5 * d151"
equation "\"d154\" = 0.5 * d153"
equation "\"d172\" = d171"
equation "\"d173\" = d172"
equation "\"d174\" = d172"
equation "\"d175\" = d173"
equation "\"d176\" = d171"
equation "\"d177\" = d170"
